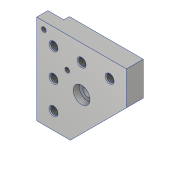
# Autodesk Inventor part: 200-20-ROCKER-CONNECTOR-04
Saved by Autodesk Inventor 2018.2 (Build 222227000, 227)
## iProperties
Manager: feesmrt
Company: FRANCOR
Part Number: 200-20-ROCKER-CONNECTOR-04
Material: Aluminium 6061
Document SubType Name: Modeling
Designer: feesmrt
Density: 2.7 g/cm^3
Appearance: Aluminium - flach
Project: Rescue Robot
Cost Center: -
Engineer: feesmrt
Authority: feesmrt
Description: Rocker Profile Connector 90°
Stock Number: 200-20-ROCKER-CONNECTOR-04
Author: feesmrt
Subject: Rescue Robot
Revision Number: 1
Title: Rocker Profile Connector 90°
Autodesk Inventor part; units mm, degrees
ref_plane "YZ Plane" through (0, 0, 0) normal (1, 0, 0) x (0, 1, 0)
ref_plane "XZ Plane" through (0, 0, 0) normal (0, 1, 0) x (-1, 0, 0)
ref_plane "XY Plane" through (0, 0, 0) normal (0, 0, 1) x (1, 0, 0)
sketch "Basisskizze" plane through (0, 0, 0) normal (0, 1, 0) x (-1, 0, 0)
  line L0 (0, -56) -> (0, 56) construction
  line L1 (56, 0) -> (-56, 0) construction
  line L2 (40, -40) -> (-40, -40)
  line L3 (-40, -40) -> (-40, 40)
  line L4 (-40, 40) -> (40, 40)
  line L5 (40, 40) -> (40, -40)
  line L6 (10, -40) -> (10, 10) construction
  line L7 (10, 10) -> (-40, 10) construction
  point P0 (0, 0)
  dimension "d2" = 80
  dimension "d3" = 30
  dimension "d4" = 30
  constraints: 12 end point, 4 perpendicular, 2 parallel, 2 point on line, 1 horizontal, 2 other
  measures "d2" distance of L3.end L4.end
  measures "d3" distance between parallel lines of L5 L6
  measures "d4" distance between parallel lines of L4 L7
extrude "Grundkörper" add sketch "Basisskizze" along normal mid plane 15
sketch "Skizze5" plane through (0, -7.5, 0) normal (0, -1, 0) x (1, 0, 0)
  line L0 (-10, -40) -> (40, 10)
  line L1 (40, 40) -> (-40, 40) projected
  line L2 (-40, 40) -> (-40, -40) projected
  line L3 (-40, -40) -> (40, -40) projected
  line L4 (40, -40) -> (40, 40) projected
  point P0 (0, 0)
  dimension "d19" = 30
  dimension "d20" = 30
  constraints: 2 end point, 2 point on line
  measures "d19" distance from line of L1 L0.end
  measures "d20" distance from line of L2 L0.start
extrude "Abschnitt" cut sketch "Skizze5" against normal through all contours L0 L4 L3
sketch "Skizze6" plane through (0, -7.5, 0) normal (0, -1, 0) x (1, 0, 0)
  line L0 (-10, -40) -> (40, 10) projected
  line L1 (-40, -40) -> (-40, 40) projected
  line L2 (15, -15) -> (-40, 40) construction
  line L3 (-40, -40) -> (-10, -40) projected
  line L4 (-10, -40) -> (-10, 40)
  line L5 (-40, 40) -> (40, 40) projected
  line L6 (40, 10) -> (-40, 10)
  point P0 (0, 0)
  point P1 (0, 0)
  dimension "d23" = 40
  dimension "d24" = 21.2132
  constraints: 6 end point, 3 point on line, 2 perpendicular, 1 midpoint, 1 vertical
  measures "d23" distance from line of point (0, 0) L3
  measures "d24" distance from line of L0 point (0, 0)
hole "DIN7984_M8" at (0, -7.5, 0) direction (0, 1, 0) diameter 9 end through all counterbore diameter 15 counterbore depth 5.4
sketch "Skizze7" plane through (0, 7.5, 0) normal (0, 1, 0) x (1, 0, 0)
  line L0 (40, -10) -> (-10, 40) construction
  line L1 (15, 15) -> (-40, -40) construction
  line L2 (22.0711, 7.9289) -> (-32.9289, -47.0711)
  line L3 (-32.9289, -47.0711) -> (-47.0711, -32.9289)
  line L4 (-47.0711, -32.9289) -> (7.9289, 22.0711)
  line L5 (7.9289, 22.0711) -> (22.0711, 7.9289)
  point P0 (0, 0)
  dimension "d32" = 20
  constraints: 10 end point, 3 perpendicular, 2 midpoint, 2 parallel, 1 coincident, 1 point on line, 1 other
  measures "d32" distance between parallel lines of L4 L2
extrude "NUT_Torsionssicherung" cut sketch "Skizze7" against normal blind 5
sketch "Skizze8" plane through (0, -7.5, 0) normal (0, -1, 0) x (1, 0, 0)
  line L0 (-10, -40) -> (-40, -40) projected
  line L1 (-25.8579, 40) -> (40, 40) projected
  line L2 (-40, 40) -> (-40, -40) projected
  line L3 (-40, 25.8579) -> (7.9289, -22.0711) projected
  line L4 (-25, -40) -> (-25, 40) construction
  line L5 (40, 40) -> (-40, 40) projected
  line L6 (-40, -40) -> (-10, -40) projected
  line L7 (40, 40) -> (40, 10) projected
  line L8 (40, 25) -> (-40, 25) construction
  line L9 (40, 10) -> (40, 40) projected
  point P0 (0, 0)
  point P1 (-25, 25)
  point P2 (-25, 0)
  point P3 (-25, -25)
  point P4 (0, 25)
  point P5 (25, 25)
  dimension "d38" = 15
  dimension "d39" = 15
  dimension "d43" = 25
  dimension "d48" = 25
  dimension "d49" = 25
  constraints: 5 point on line, 4 end point, 3 midpoint, 2 perpendicular, 1 vertical, 2 other
  measures "d38" distance between parallel lines of L2 L4
  measures "d39" distance between parallel lines of L1 L8
  measures "d43" distance of point (-25, 25) point (-25, 0)
  measures "d48" distance of point (-25, 25) point (0, 25)
  measures "d49" distance of point (25, 25) point (0, 25)
hole "M8_Profilgewinde" at (-25, -7.5, 25) at (-25, -7.5, 0) at (-25, -7.5, -25) at (0, -7.5, 25) at (25, -7.5, 25) direction (0, 1, 0) diameter 6.647 end through all countersink diameter 8 countersink angle 90 thread size "M8x1.25" class "6H" standard "ISO Metric profile"
sketch "Skizze9" plane through (0, 2.5, 0) normal (0, 1, 0) x (1, 0, 0)
  circle A0 centre (-25, -25) radius 3.3235 construction
  circle A1 centre (0, 0) radius 4.5 construction
  line L0 (40, -40) -> (-40, -40) projected
  line L1 (-40, -40) -> (0, 0) construction
  line L2 (-17.9289, -32.0711) -> (-32.0711, -17.9289) construction
  line L3 (-40, -25.8579) -> (7.9289, 22.0711) projected
  line L4 (22.0711, 7.9289) -> (-25.8579, -40) projected
  line L5 (-40, 40) -> (-40, -25.8579) projected
  line L6 (7.9289, 22.0711) -> (22.0711, 7.9289) projected
  point P0 (0, 0)
  point P1 (-12.7279, -12.7279)
  point P2 (-33.5876, -33.5876)
  dimension "d72" = 18
  dimension "d73" = 47.5
  constraints: 4 end point, 4 point on line, 1 midpoint, 1 perpendicular
  measures "d72" distance of point (-12.728, -12.728) point (0, 0)
  measures "d73" distance of point (-33.588, -33.588) point (0, 0)
hole "M5_Bohrung" at (-12.7279, 2.5, 12.7279) at (-33.5876, 2.5, 33.5876) direction (0, -1, 0) diameter 4.134 end through all countersink diameter 5 countersink angle 90 thread size "M5x0.8" class "6H" standard "ISO Metric profile"
equation "\"d4\" = d3"
equation "\"d48\" = d43"
equation "\"d49\" = d48"
